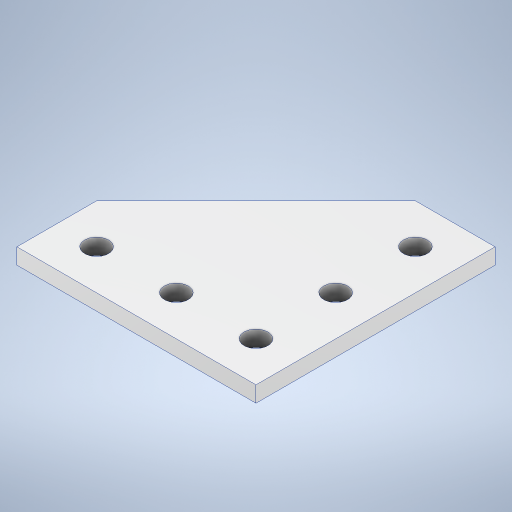
# Autodesk Inventor part: corner_bracket
Saved by Autodesk Inventor 2024 (Build 280153000, 153)
## iProperties
Created: 2024-09-20
Part Number: corner_bracket
Material: Aluminum 6061
Document SubType Name: Modeling
Designer: Owner
Density: 2.7 g/cm^3
Appearance: Aluminum - Flat
Author: Owner
Autodesk Inventor part; units mm, degrees
ref_plane "YZ Plane" through (0, 0, 0) normal (1, 0, 0) x (0, 1, 0)
ref_plane "XZ Plane" through (0, 0, 0) normal (0, 1, 0) x (-1, 0, 0)
ref_plane "XY Plane" through (0, 0, 0) normal (0, 0, 1) x (1, 0, 0)
sketch "Sketch1" plane through (0, 0, 0) normal (0, 1, 0) x (-1, 0, 0)
  line L0 (0, 0) -> (25.4, 0)
  line L1 (25.4, 0) -> (25.4, -76.2)
  line L2 (25.4, -76.2) -> (0, -76.2)
  line L3 (0, -76.2) -> (0, 0)
  line L4 (0, 0) -> (76.2, 0)
  line L5 (76.2, 0) -> (76.2, -25.4)
  line L6 (76.2, -25.4) -> (0, -25.4)
  line L7 (0, -25.4) -> (0, 0)
  line L8 (76.2, -12.7) -> (0, -12.7)
  line L9 (12.7, -76.2) -> (12.7, 0)
  line L10 (12.7, -12.7) -> (38.1, -12.7)
  line L11 (38.1, -12.7) -> (63.5, -12.7)
  line L12 (12.7, -12.7) -> (12.7, -38.1)
  line L13 (12.7, -38.1) -> (12.7, -63.5)
  circle A0 centre (12.7, -12.7) radius 3.81
  circle A1 centre (38.1, -12.7) radius 3.81
  circle A2 centre (63.5, -12.7) radius 3.81
  circle A3 centre (12.7, -38.1) radius 3.81
  circle A4 centre (12.7, -63.5) radius 3.81
  line L14 (76.2, -25.4) -> (25.4, -76.2)
  point P0 (25.4, -25.4)
  dimension "d0" = 25.4
  dimension "d1" = 76.2
  dimension "d2" = 76.2
  dimension "d3" = 25.4
  dimension "d4" = 25.4
  dimension "d5" = 25.4
  dimension "d6" = 25.4
  dimension "d7" = 25.4
  dimension "d8" = 7.62
  dimension "d9" = 7.62
  dimension "d10" = 7.62
  dimension "d11" = 7.62
  dimension "d12" = 7.62
  constraints: 30 end point, 5 centre point, 5 coincident, 5 midpoint, 5 point on line, 4 parallel, 3 perpendicular, 2 horizontal
  measures "d0" distance of L1.end L2.end
  measures "d1" distance of L0.end L1.end
  measures "d2" distance of L5.end L6.end
  measures "d3" distance of L4.end L5.end
  measures "d4" distance of L10.start L10.end
  measures "d5" distance of L10.end L11.end
  measures "d6" distance of L10.start L12.end
  measures "d7" distance of L12.end L13.end
  measures "d8" diameter of A0
  measures "d9" diameter of A1
  measures "d10" diameter of A2
  measures "d11" diameter of A3
  measures "d12" diameter of A4
extrude "Extrusion1" add sketch "Sketch1" along normal blind 5.08 contours L0 L9 A0 L8 L3 | L0 L1 L8 A0 L9 | L8 A0 L9 L6 L3 | L4 L5 L8 A2 A1 L1 | L6 L9 A3 A4 L2 L3 | L8 A1 A2 L5 L6 L1 | L1 L6 L9 A0 L8 | L6 L1 L2 L9 A4 A3 | L6 L14 L1
equation "\"d9\" = d8"
equation "\"d10\" = d8"
equation "\"d11\" = d8"
equation "\"d12\" = d8"
body "Solid1"
